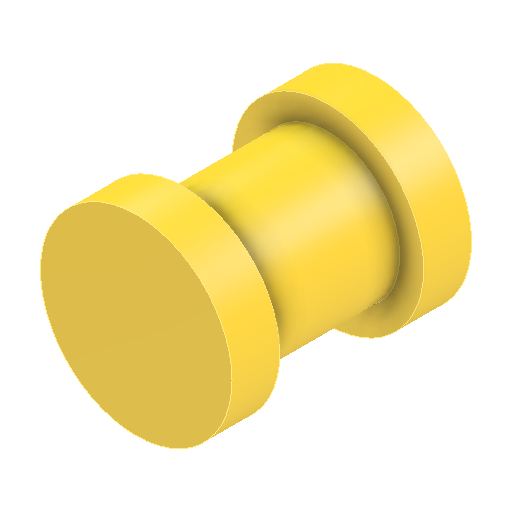
# Autodesk Inventor part: 00_Threaded_Screw_Insert_M3
Saved by Autodesk Inventor 2022 (Build 260153000, 153)
## iProperties
Created: 2022-09-25
Part Number: 00_Threaded_Screw_Insert_M3
Material: Generisch
Document SubType Name: Modeling
Designer: UC2
Density: 1 g/cm^3
Appearance: Glänzend - Gold
Catalog Web Link: https://detail.tmall.com/item_o.htm?id=642445155037&spm=a1z09.2.0.0.366c2e8dELQBXu&_u=d1hhfjuvbb45
Vendor: Taobao
Author: UC2
Autodesk Inventor part; units mm, degrees
ref_plane "YZ Plane" through (0, 0, 0) normal (1, 0, 0) x (0, 1, 0)
ref_plane "XZ Plane" through (0, 0, 0) normal (0, 1, 0) x (-1, 0, 0)
ref_plane "XY Plane" through (0, 0, 0) normal (0, 0, 1) x (1, 0, 0)
sketch "Skizze1" plane through (0, 0, 0) normal (0, 1, 0) x (-1, 0, 0)
  line L0 (0, 0) -> (0, -5)
  line L1 (0, -5) -> (2, -5)
  line L2 (2, -5) -> (2, -4)
  line L3 (2, -4) -> (1.5, -4)
  line L4 (1.5, -4) -> (1.5, -1)
  line L5 (1.5, -1) -> (2, -1)
  line L6 (2, -1) -> (2, 0)
  line L7 (2, 0) -> (0, 0)
  dimension "d0" = 5
  dimension "d1" = 1
  dimension "d2" = 0.5
  dimension "d3" = 1
  dimension "d5" = 2
  constraints: 16 end point, 6 perpendicular, 2 point on line, 1 vertical
  measures "d0" distance of L0.start L0.end
  measures "d1" distance of L1.end L2.end
  measures "d2" distance of L2.end L3.end
  measures "d3" distance between parallel lines of L7 L5
  measures "d5" distance between parallel lines of L0 L2
revolve "Umdrehung1" add sketch "Skizze1" angle 360 about axis through (0, 0, 0) along (0, 0, -1)
